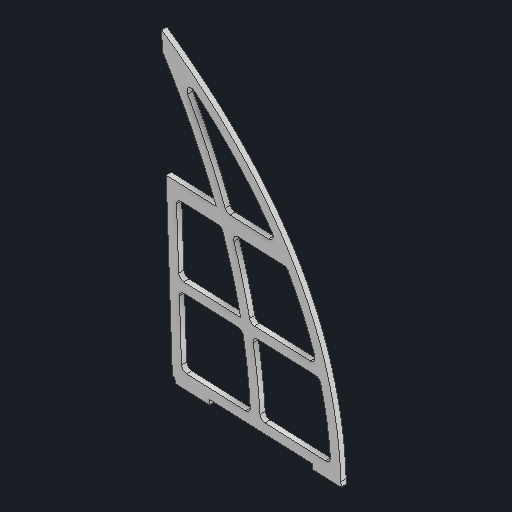
# Autodesk Inventor part: sponson_spanner_side
Saved by Autodesk Inventor 2023 (Build 270158030, 158C)
## iProperties
Created: 2022-03-22
Part Number: sponson_spanner_side
Material: Generic
Document SubType Name: Modeling
Designer: kardo
Density: 1 g/cm^3
Appearance: Default
Author: kardo
Autodesk Inventor part; units mm, degrees
ref_plane "YZ Plane" through (0, 0, 0) normal (1, 0, 0) x (0, 1, 0)
ref_plane "XZ Plane" through (0, 0, 0) normal (0, 1, 0) x (-1, 0, 0)
ref_plane "XY Plane" through (0, 0, 0) normal (0, 0, 1) x (1, 0, 0)
derived "surface_body.ipt"
sketch "sk_rail_sponson_side" plane through (81.12, 237, 36.448) normal (0.0378267, 0.0348745, -0.9986756) x (0.3011979, -0.9533106, -0.0218819)
  line L0 (248.6073, 0) -> (144.1371, -33.0246)
  spline S0 degree 2 poles (144.1371, -33.0246) (68.7786, -56.8465) (0, 0) knots 0 0 0 1 1 1
  point P0 (202.299, 150.0824)
ref_plane "plane_tunnel_right" through (81.12, 0, 0) normal (1, 0, 0) x (0, 1, 0)
ref_plane "plane_sponson_side" through (81.12, 237, 36.448) normal (0.0378267, 0.0348745, -0.9986756) x (0.3011979, -0.9533106, -0.0218819)
sketch "sk_rail_sponson_tunnel" plane through (81.12, 0, 0) normal (1, 0, 0) x (0, 1, 0)
  line L0 (0, 0) -> (111.39, 7.7891)
  line L1 (101.5485, 148.5297) -> (128.7646, -240.679) construction
  spline S0 degree 2 poles (111.39, 7.7891) (176.0348, 12.3096) (237, 36.448) knots 0 0 0 1 1 1
sketch "sk_rail_sponson_bottom" plane through (126.048, 0, 0) normal (0.4037383, -0.0638184, 0.9126459) x (-0.1841621, 0.9714748, 0.1494022)
  line L0 (109.3763, -22.4773) -> (0, 0)
  line L1 (371.255, -76.2945) -> (-489.8119, 100.6585) construction
  line L2 (156.3866, 206.2785) -> (76.3238, -183.3132) construction
  spline S0 degree 2 poles (109.3763, -22.4773) (178.4423, -36.6707) (243.959, 0) knots 0 0 0 1 1 1
  point P0 (23.2133, 112.9576)
sketch "sk_rail_top_tunnel" plane through (81.12, 0, 0) normal (1, 0, 0) x (0, 1, 0)
  line L0 (237, 107.6209) -> (237, -224.5198) construction
  line L1 (0, 107.6209) -> (0, -224.5198) construction
  line L2 (-363, 107.6209) -> (-363, -224.5198) construction
  line L3 (-363, 0) -> (0, 0) construction
  line L4 (-181.5, 48.8998) -> (-181.5, 0) construction
  line L5 (0, 52.89) -> (52.14, 52.89) construction
  line L6 (52.14, 52.89) -> (75.84, 48.2838) construction
  line L7 (75.84, 48.2838) -> (94.8, 37.536) construction
  line L8 (94.8, 107.6209) -> (94.8, -224.5198) construction
  line L9 (0, 52.89) -> (237, 52.89) construction
  line L10 (-488.1035, 0) -> (361.1125, 0) construction
  spline S0 degree 3 poles (0, 52.89) (86.3106, 52.89) (181.3207, 49.5034) (237, 36.448) knots 0 0 0 0 1 1 1 1
  spline S1 degree 3 poles (0, 52.89) (52.14, 52.89) (75.84, 48.2838) (94.8, 37.536) knots 1 1 1 1 2 2 2 2
  spline S2 degree 4 poles (-363, 37.4293) (-272.3626, 45.1427) (-181.5879, 49.7528) (-90.8131, 52.89) (0, 52.89) knots 0 0 0 0 0 1 1 1 1 1
  point P0 (142.2, 48.7795)
  point P1 (94.8, 28.832)
  point P2 (-242.0001, 45.8501)
  point P3 (-120.9999, 51.0063)
sketch "sk_section_sponson_break" plane through (0, 111.39, 7.7891) normal (0, 0.9975641, 0.0697565) x (-1, 0, 0)
  line L0 (-276.1283, -66.2311) -> (62.1846, 83.0679) construction
  line L1 (-81.12, -261.3468) -> (-81.12, 152.2132) construction
  arc A0 (-81.12, 43.0127) -> (-156, 27.1087) centre (-69.8132, -194.4509) ccw construction
  arc A1 (-54.6, 54.2675) -> (-156, 30.9325) centre (-53.2768, -183.4615) ccw construction
  spline S0 degree 2 poles (-54.6, 54.2675) (-107.2974, 54.2675) (-156, 30.9325) knots 0 0 0 1 1 1
  spline S1 degree 2 poles (-156, 27.1087) (-120.096, 41.0753) (-81.12, 43.0127) knots 0 0 0 1 1 1
  point P0 (0, 0)
ref_plane "plane_sponson_break" through (0, 111.39, 7.7891) normal (0, 0.9975641, 0.0697565) x (-1, 0, 0)
derived "parameters_frame.ipt"
derived "stencil_frame.ipt"
sketch "sk_joint_locations" plane through (81.12, 0, 0) normal (1, 0, 0) x (0, 1, 0)
  line L0 (0, 0) -> (111.39, 7.7891) construction
  line L1 (30.81, 28.832) -> (94.8, 28.832) construction
  arc A0 (30.81, 28.832) -> (9.48, 28.4869) centre (30.81, -630.4631) ccw construction
  line L2 (-254.1001, 19.9549) -> (9.48, 28.4869) construction
  line L3 (-363, 18.496) -> (-275.8801, 19.4795) construction
  arc A1 (-275.8801, 19.4795) -> (-254.1001, 19.9549) centre (-287.5515, 1053.3708) ccw construction
  line L4 (1.436, 1580.2049) -> (243.9436, -1887.8151) construction
  line L5 (-242.0001, 1541.8302) -> (-242.0001, -1877.3857) construction
  line L6 (-120.9999, 1541.8302) -> (-120.9999, -1877.3857) construction
  line L7 (-363, 1541.8302) -> (-363, -1877.3857) construction
  line L8 (0, 1541.8302) -> (0, -1877.3857) construction
  line L9 (445.406, 43.7257) -> (-613.1443, 6.7603) construction
  line L10 (-676.709, -27.4448) -> (497.0858, 54.635) construction
  line L11 (178.2183, 30.3929) -> (177.9391, 38.388) construction
  line L12 (185.9231, 36.8959) -> (186.4825, 28.8959) construction
  line L13 (0, 6.528) -> (111.1168, 11.6964) construction
  line L14 (-242.0001, 45.8501) -> (-242.0001, 20.3465) construction
  line L15 (-363, 37.4293) -> (-363, 18.496) construction
  line L16 (-120.9999, 51.0063) -> (-120.9999, 24.2633) construction
  line L17 (0, 52.89) -> (0, 28.18) construction
  line L18 (108.3896, 50.6971) -> (108.935, 42.897) construction
  line L19 (109.4805, 35.0968) -> (108.935, 42.897) construction
  line L20 (109.4805, 35.0968) -> (110.0259, 27.2967) construction
  line L21 (110.0259, 27.2967) -> (110.5713, 19.4965) construction
  line L22 (110.5713, 19.4965) -> (111.1168, 11.6964) construction
  line L23 (0, 6.528) -> (0, 0) construction
  line L24 (94.8, 37.536) -> (94.8, 28.832) construction
  line L25 (94.8, 35.548) -> (94.8, 30.82) construction
  spline S0 degree 4 poles (-363, 37.4293) (-272.3626, 45.1427) (-181.5879, 49.7528) (-90.8131, 52.89) (0, 52.89) knots 0 0 0 0 0 1 1 1 1 1
  spline S1 degree 3 poles (0, 52.89) (86.3106, 52.89) (181.3207, 49.5034) (237, 36.448) knots 0 0 0 0 1 1 1 1
  spline S2 degree 2 poles (111.39, 7.7891) (176.0348, 12.3096) (237, 36.448) knots 0 0 0 1 1 1
  point P0 (1.436, 1580.2049)
  point P1 (243.9436, -1887.8151)
  point P2 (178.0787, 34.3904)
  point P3 (186.2028, 32.8959)
  point P4 (134.9575, 11.3411)
  point P5 (-363, 27.9627)
  point P6 (-242.0001, 33.0983)
  point P7 (-120.9999, 37.6348)
  point P8 (0, 40.535)
  point P9 (94.8, 33.184)
sketch "sk_spanner_joints_locations" plane through (0, 111.39, 7.7891) normal (0, 0.9975641, 0.0697565) x (-1, 0, 0)
  line L0 (280.557, 10.5733) -> (-334.5102, 33.8701) construction
  line L1 (-953.5208, -365.1675) -> (735.9219, 380.3912) construction
  line L2 (-85.1788, 24.4262) -> (-84.0523, 18.5329) construction
  line L3 (-85.1788, 24.4262) -> (-71.8427, 23.9211) construction
  line L4 (-84.0523, 18.5329) -> (-71.8427, 23.9211) construction
  point P0 (0, 0)
  point P1 (-126.048, 0)
  point P2 (-156, 27.1087)
  point P3 (-141.8358, 26.5722)
  point P4 (-99.343, 24.9627)
  point P5 (-94.5512, 13.8997)
  point P6 (-115.5491, 4.6332)
ref_plane "plane_stringer_outer" through (84.12, 0, 0) normal (1, 0, 0) x (0, 1, 0)
sketch "sk_corner_offset" plane through (0, 111.39, 7.7891) normal (0, 0.9975641, 0.0697565) x (-1, 0, 0)
  spline S0 degree 2 poles (-156, 27.1087) (-120.096, 41.0753) (-81.12, 43.0127) knots 0 0 0 1 1 1 construction
  line L0 (-156, 27.1087) -> (-126.048, 0) construction
  line L1 (-153.7477, 26.6887) -> (-125.2428, 0.8897) construction
  line L2 (-125.2428, 0.8897) -> (-126.048, 0) construction
  spline S1 degree 5 poles (-153.7477, 26.6887) (-139.8082, 31.9809) (-125.456, 36.1868) (-110.7888, 39.2205) (-95.9524, 41.0738) (-81.0604, 41.8142) knots 0 0 0 0 0 0 1 1 1 1 1 1 construction
  point P0 (0, 0)
  dimension "d9" = 1.2
  dimension "d10" = 1.2
  constraints: 6 end point, 1 coincident, 1 parallel, 1 perpendicular, 3 other
  measures "d10" distance between parallel lines of L1 L0
sketch "sk_tip_offset" plane through (81.12, 0, 0) normal (1, 0, 0) x (0, 1, 0)
  spline S0 degree 3 poles (0, 52.89) (86.3106, 52.89) (181.3207, 49.5034) (237, 36.448) knots 0 0 0 0 1 1 1 1 construction
  spline S1 degree 2 poles (111.39, 7.7891) (176.0348, 12.3096) (237, 36.448) knots 0 0 0 1 1 1 construction
  spline S2 degree 5 poles (0, 51.69) (13.1181, 51.69) (26.2363, 51.6248) (39.354, 51.4874) (65.3463, 51.0551) (91.3298, 50.254) (104.1978, 49.754) (128.8047, 48.5691) (153.3792, 46.8416) (165.0971, 45.8705) (185.7675, 43.844) (206.3487, 41.0607) (215.2522, 39.6762) (224.1241, 38.0772) (232.9228, 36.143) knots 0 0 0 0 0 0 0.280538 0.280538 0.280538 0.555921 0.555921 0.555921 0.807344 0.807344 0.807344 1 1 1 1 1 1 construction
  spline S3 degree 5 poles (111.3063, 8.9862) (136.261, 10.7315) (161.0871, 14.3225) (185.5959, 19.817) (209.5823, 27.1424) (232.9228, 36.1431) knots 0 0 0 0 0 0 1 1 1 1 1 1 construction
  point P0 (0, 0)
  dimension "d7" = 1.2
  dimension "d8" = 1.2
  constraints: 1 coincident, 6 other
sketch "sk_sponson_spanner_side_base" plane through (81.12, 237, 36.448) normal (0.0378267, 0.0348745, -0.9986756) x (0.3011979, -0.9533106, -0.0218819)
  spline S0 degree 2 poles (144.1371, -33.0246) (68.7786, -56.8465) (0, 0) knots 0 0 0 1 1 1 construction
  line L0 (122.6861, 34.5231) -> (122.3654, 35.533)
  line L1 (126.9763, 21.0136) -> (139.8469, -19.5151)
  line L2 (139.8469, -19.5151) -> (141.7531, -18.9097)
  line L3 (141.7531, -18.9097) -> (145.3581, -30.2615)
  line L4 (126.9763, 21.0136) -> (128.8825, 21.6189)
  line L5 (128.8825, 21.6189) -> (124.5923, 35.1284)
  line L6 (124.5923, 35.1284) -> (122.6861, 34.5231)
  line L7 (728.8749, 227.2597) -> (-184.0748, -61.3374) projected
  line L8 (145.3581, -30.2615) -> (143.44, -30.8679)
  line L9 (248.6073, 0) -> (144.1371, -33.0246) construction
  spline S1 degree 2 poles (3.8935, 1.2373) (70.4509, -53.9408) (143.44, -30.8679) knots 0 0 0 1 1 1
  point P0 (202.299, 150.0824)
  point P1 (144.1371, -33.0246)
  point P2 (56.2153, 17.7705)
  point P3 (99.6986, 28.3676)
  point P4 (2.7864, -2.2678)
  point P5 (6.6806, -1.0367)
  dimension "d3" = 2
  constraints: 16 end point, 4 parallel, 2 collinear, 2 perpendicular, 1 point on line, 3 other
  measures "d3" distance between parallel lines of L5 L1
extrude "thicken" add sketch "sk_sponson_spanner_side_base" along normal blind 2
sketch "sk_cut_weight" plane through (81.12, 237, 36.448) normal (0.0378267, 0.0348745, -0.9986756) x (0.3011979, -0.9533106, -0.0218819)
  line L0 (122.6861, 34.5231) -> (122.3654, 35.533) construction
  line L1 (126.9763, 21.0136) -> (139.8469, -19.5151) construction
  spline S0 degree 2 poles (3.8935, 1.2373) (70.4509, -53.9408) (143.44, -30.8679) knots 0 0 0 1 1 1 construction
  line L2 (56.2153, 17.7705) -> (71.3476, -30.099) construction
  line L3 (62.1398, 12.2996) -> (67.7709, -5.5139)
  line L4 (55.2132, 14.3051) -> (61.4477, -5.4171)
  line L5 (55.2132, 14.3051) -> (13.8505, 1.2298)
  line L6 (62.1398, 12.2996) -> (119.7621, 30.5149)
  line L7 (119.7621, 30.5149) -> (128.3777, 3.385)
  line L8 (69.0344, -9.5107) -> (75.8633, -31.1132)
  line L9 (62.7235, -9.4529) -> (69.0674, -29.5213)
  line L10 (129.5886, -0.428) -> (138.4109, -28.2088)
  line L11 (90.951, 21.4073) -> (108.2944, -33.4571) construction
  line L12 (96.732, -3.5159) -> (89.044, 20.8045)
  line L13 (92.8579, 22.0101) -> (100.7382, -2.9185)
  line L14 (101.9571, -6.7741) -> (110.3489, -33.321)
  line L15 (97.9545, -7.3831) -> (106.2295, -33.5605)
  line L16 (728.8749, 227.2597) -> (-184.0748, -61.3374) construction
  spline S1 degree 2 poles (133.4116, 0.7492) (71.7217, -18.8415) (6.6806, -1.0367) knots 0 0 0 1 1 1
  spline S2 degree 5 poles (16.4601, -3.5068) (22.8185, -8.173) (29.4037, -12.5301) (36.2231, -16.5261) (51.6054, -24.3076) (67.9783, -29.7458) (77.0955, -31.8969) (94.9737, -34.3408) (112.9891, -33.541) (121.61, -32.4078) (130.0951, -30.6034) (138.4109, -28.2088) knots 0 0 0 0 0 0 0.305076 0.305076 0.305076 0.665259 0.665259 0.665259 1 1 1 1 1 1
  spline S3 degree 5 poles (128.3777, 3.385) (117.1808, 0.0489) (105.7646, -2.551) (94.1806, -4.3536) (71.0161, -6.2884) (47.8065, -5.0315) (36.3519, -3.6367) (25.0211, -1.5279) (13.8505, 1.2298) knots 0 0 0 0 0 0 0.503823 0.503823 0.503823 1 1 1 1 1 1
  point P0 (202.299, 150.0824)
  dimension "d11" = 4
  dimension "d20" = 4
  dimension "d14" = 2
  dimension "d15" = 4
  dimension "d16" = 4
  dimension "d19" = 4
  dimension "d21" = 4
  constraints: 28 end point, 6 collinear, 5 parallel, 3 point on line, 2 midpoint, 2 perpendicular, 28 other
  measures "d14" distance between parallel lines of L2 L4
  measures "d15" distance between parallel lines of L2 L3
  measures "d16" distance between parallel lines of L1 L7
  measures "d19" distance between parallel lines of L13 L12
  measures "d21" distance between parallel lines of L16 L6
extrude "cut_weight" cut sketch "sk_cut_weight" along normal through all both and the other way through all contours L6 L12 S3 L3 | L6 L7 S3 L13 | L4 S3 L5 | S1 L15 S2 L8 | L9 S2 S1 | S1 L10 S2 L14
fillet "rounding" radius 2 18 edges at (88.155, 113.7108, 31.4078) (120.5974, 113.6251, 32.6336) (117.6962, 145.8686, 33.6497) (88.155, 145.9076, 32.5321) (109.0568, 180.0755, 34.517) (88.155, 141.91, 32.3925) (88.155, 174.1068, 33.5169) (111.0128, 174.0766, 34.3816) (89.4569, 222.3953, 35.2524) (118.3215, 141.8702, 33.5337) (106.824, 174.0821, 34.2231) (133.6527, 174.0467, 35.2381) (114.2807, 141.8755, 33.3809) (146.1433, 141.8334, 34.5863) (130.089, 180.0477, 35.3127) (149.7245, 113.5481, 33.7342) (145.1307, 145.8323, 34.6876) (116.5996, 113.6356, 32.4826)
equation "\"d9\" = shell_thickness"
equation "\"d10\" = shell_thickness"
equation "\"d7\" = shell_thickness"
equation "\"d8\" = shell_thickness"
equation "\"d3\" = bulkhead_thickness"
equation "\"d5\" = bulkhead_thickness"
equation "\"d11\" = bulkhead_inset"
equation "\"d20\" = bulkhead_inset"
equation "\"d14\" = bulkhead_thickness"
equation "\"d15\" = 2 * bulkhead_thickness"
equation "\"d16\" = bulkhead_inset"
equation "\"d19\" = bulkhead_inset"
equation "\"d21\" = bulkhead_inset"
equation "\"d25\" = 0.5 * bulkhead_inset"
equation "\"d4\" = stringer_thickness"
equation "\"shell_thickness\" = 1.2"
equation "\"bulkhead_thickness\" = 2"
equation "\"bulkhead_inset\" = 4"
equation "\"stringer_thickness\" = 3"
body "Solid1"
